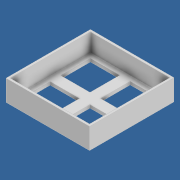
# Autodesk Inventor part: test plate
Saved by Autodesk Inventor 2020 (Build 240168000, 168)
## iProperties
Created: 2021-09-04
Part Number: test plate
Material: Generic
Document SubType Name: Modeling
Designer: RNG3nius
Density: 1 g/cm^3
Appearance: Default
Author: RNG3nius
Autodesk Inventor part; units mm, degrees
ref_plane "YZ Plane" through (0, 0, 0) normal (1, 0, 0) x (0, 1, 0)
ref_plane "XZ Plane" through (0, 0, 0) normal (0, 1, 0) x (-1, 0, 0)
ref_plane "XY Plane" through (0, 0, 0) normal (0, 0, 1) x (1, 0, 0)
sketch "Sketch1" plane through (0, 0, 0) normal (0, 1, 0) x (-1, 0, 0)
  line L0 (0, 0) -> (39.9, 0)
  line L1 (39.9, 0) -> (39.9, 40.3)
  line L2 (39.9, 40.3) -> (0, 40.3)
  line L3 (0, 40.3) -> (0, 0)
  dimension "d0" = 39.9
  dimension "d1" = 40.3
  constraints: 8 end point, 2 parallel, 1 horizontal, 1 perpendicular
  measures "d0" distance of L2.end L1.end
  measures "d1" distance of L1.end L0.end
extrude "Extrusion1" add sketch "Sketch1" along normal blind 10
sketch "Sketch8" plane through (0, 10, 0) normal (0, 1, 0) x (1, 0, 0)
  line L0 (-1, -1) -> (-38.9, -1)
  line L1 (-38.9, -1) -> (-38.9, -39.3)
  line L2 (-38.9, -39.3) -> (-1, -39.3)
  line L3 (-1, -39.3) -> (-1, -1)
  line L4 (0, 0) -> (-39.9, 0) projected
  line L5 (0, -40.3) -> (0, 0) projected
  dimension "d61" = 37.9
  dimension "d62" = 38.3
  dimension "d63" = 1
  dimension "d64" = 1
  constraints: 8 end point, 2 parallel, 1 horizontal, 1 perpendicular
  measures "d61" distance of L2.end L1.end
  measures "d62" distance of L1.end L0.end
  measures "d63" distance between parallel lines of L4 L0
  measures "d64" distance between parallel lines of L5 L3
extrude "Extrusion7" cut sketch "Sketch8" against normal blind 8.5
sketch "Sketch9" plane through (0, 1.5, 0) normal (0, 1, 0) x (1, 0, 0)
  line L0 (-3.45, -3.45) -> (-17.45, -3.45)
  line L1 (-17.45, -3.45) -> (-17.45, -17.65)
  line L2 (-17.45, -17.65) -> (-3.45, -17.65)
  line L3 (-3.45, -17.65) -> (-3.45, -3.45)
  line L4 (-1, -1) -> (-1, -39.3) projected
  line L5 (-38.9, -1) -> (-1, -1) projected
  line L6 (-22.45, -3.45) -> (-36.45, -3.45)
  line L7 (-36.45, -3.45) -> (-36.45, -17.65)
  line L8 (-36.45, -17.65) -> (-22.45, -17.65)
  line L9 (-22.45, -17.65) -> (-22.45, -3.45)
  line L10 (-22.45, -22.65) -> (-36.45, -22.65)
  line L11 (-36.45, -22.65) -> (-36.45, -36.85)
  line L12 (-36.45, -36.85) -> (-22.45, -36.85)
  line L13 (-22.45, -36.85) -> (-22.45, -22.65)
  line L14 (-38.9, -39.3) -> (-38.9, -1) projected
  line L15 (-17.45, -22.65) -> (-3.45, -22.65)
  line L16 (-3.45, -22.65) -> (-3.45, -36.85)
  line L17 (-3.45, -36.85) -> (-17.45, -36.85)
  line L18 (-17.45, -36.85) -> (-17.45, -22.65)
  point P0 (0, 0)
  dimension "d67" = 14
  dimension "d68" = 14.2
  dimension "d69" = 2.45
  dimension "d70" = 2.45
  dimension "d71" = 14
  dimension "d72" = 14.2
  dimension "d73" = 5
  dimension "d74" = 14
  dimension "d75" = 14.2
  dimension "d76" = 5
  dimension "d77" = 2.45
  dimension "d78" = 14
  dimension "d79" = 14.2
  dimension "d80" = 5
  dimension "d81" = 5
  constraints: 32 end point, 8 parallel, 4 horizontal, 4 perpendicular, 1 point on line
  measures "d67" distance of L2.end L1.end
  measures "d68" distance of L1.end L0.end
  measures "d69" distance between parallel lines of L3 L4
  measures "d70" distance between parallel lines of L5 L0
  measures "d71" distance of L8.end L7.end
  measures "d72" distance of L7.end L6.end
  measures "d73" distance between parallel lines of L9 L1
  measures "d74" distance of L12.end L11.end
  measures "d75" distance of L11.end L10.end
  measures "d76" distance between parallel lines of L8 L10
  measures "d77" distance between parallel lines of L14 L11
  measures "d78" distance of L16.end L17.end
  measures "d79" distance of L15.end L16.end
  measures "d80" distance between parallel lines of L13 L18
  measures "d81" distance between parallel lines of L2 L15
extrude "Extrusion8" cut sketch "Sketch9" against normal blind 8.5
body "Solid1"
